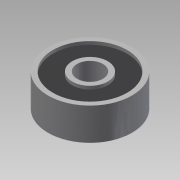
# Autodesk Inventor part: Roulement
Saved by Autodesk Inventor 2016 (Build 200138000, 138)
## iProperties
Created: 2016-01-22
Part Number: Roulement
Material: Acier
Document SubType Name: Modeling
Designer: sd
Density: 7.85 g/cm^3
Appearance: Acier
Author: sd
Autodesk Inventor part; units mm, degrees
ref_plane "YZ Plane" through (0, 0, 0) normal (1, 0, 0) x (0, 1, 0)
ref_plane "XZ Plane" through (0, 0, 0) normal (0, 1, 0) x (-1, 0, 0)
ref_plane "XY Plane" through (0, 0, 0) normal (0, 0, 1) x (1, 0, 0)
sketch "Esquisse1" plane through (0, 0, 0) normal (0, 0, 1) x (1, 0, 0)
  circle A0 centre (0, 0) radius 2
  circle A1 centre (0, 0) radius 6.5
  dimension "d0" = 4
  dimension "d1" = 13
  constraints: 2 centre point, 2 coincident
  measures "d0" diameter of A0
  measures "d1" diameter of A1
extrude "Extrusion1" add sketch "Esquisse1" along normal blind 5
sketch "Esquisse2" plane through (0, 0, 5) normal (0, 0, 1) x (1, 0, 0)
  circle A0 centre (0, 0) radius 2 projected
  circle A1 centre (0, 0) radius 6.5 projected
  circle A2 centre (0, 0) radius 2.75
  circle A3 centre (0, 0) radius 5.75
  dimension "d4" = 11.5
  dimension "d5" = 13
  dimension "d6" = 4
  dimension "d7" = 5.5
  constraints: 2 centre point, 2 coincident
  measures "d4" diameter of A3
  measures "d5" diameter of A1
  measures "d6" diameter of A0
  measures "d7" diameter of A2
extrude "Extrusion2" cut sketch "Esquisse2" against normal blind 0.5 contours A3
sketch "Esquisse3" plane through (0, 0, 0) normal (0, 0, -1) x (-1, 0, 0)
  circle A0 centre (0, 0) radius 2 projected
  circle A1 centre (0, 0) radius 6.5 projected
  circle A2 centre (0, 0) radius 2.75
  circle A3 centre (0, 0) radius 5.75
  dimension "d12" = 11.5
  dimension "d13" = 13
  dimension "d14" = 4
  dimension "d15" = 5.5
  constraints: 2 centre point, 2 coincident
  measures "d12" diameter of A3
  measures "d13" diameter of A1
  measures "d14" diameter of A0
  measures "d15" diameter of A2
extrude "Extrusion3" cut sketch "Esquisse3" against normal blind 0.5 contours A3
